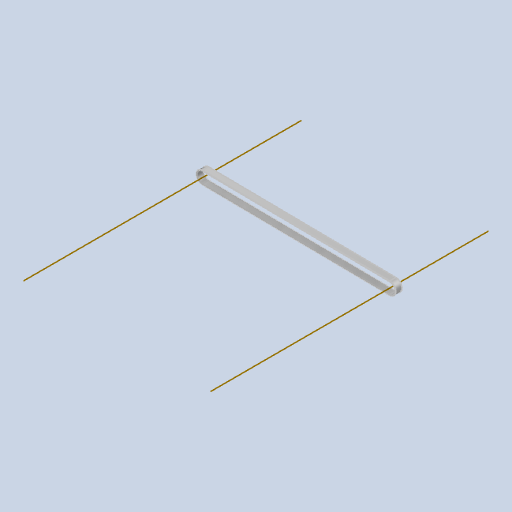
# Autodesk Inventor part: Synchronous Belt
Saved by Autodesk Inventor 2023 (Build 270158000, 158)
## iProperties
Created: 2022-10-18
Part Number: Synchronous Belt
Material: Rubber
Document SubType Name: Modeling
Designer: klebe
Density: 1 g/cm^3
Appearance: Rubber - Black - Version 1.1
CustomPartVersion: 1
Author: klebe
Autodesk Inventor part; units mm, degrees
sketch "Sketch Path" plane through (0, 0, 0) normal (0, 0, 1) x (1, 0, 0)
  arc A0 (0.0703, 6.0634) -> (-0.0703, -6.0634) centre (0, 0) ccw
  arc A1 (196.5726, -8.3439) -> (196.7132, 3.7829) centre (196.6429, -2.2805) ccw
  line L0 (196.5726, -8.3439) -> (-0.0703, -6.0634)
  line L1 (0.0703, 6.0634) -> (196.7132, 3.7829)
  constraints: 4 end point, 2 point on circle, 1 centre point, 3 other
ref_plane "Cross Section Plane" through (-0.0703, -6.0634, 0) normal (0.9999, -0.0116, 0) x (0, 0, 1)
ref_plane "Work Plane2" through (0, 0, 0) normal (-1, 0, 0) x (0, 0, 1)
ref_plane "Work Plane3" through (196.6429, -2.2805, 0) normal (-0.9995, 0.032, 0) x (0, 0, 1)
sketch "Cross Section" plane through (-0.0703, -6.0634, 0) normal (0.9999, -0.0116, 0) x (0, 0, 1)
  line L0 (-3.175, 0.508) -> (3.175, 0.508)
  line L1 (3.175, 0.508) -> (3.175, -0.254)
  line L2 (3.175, -0.254) -> (-3.175, -0.254)
  line L3 (-3.175, -0.254) -> (-3.175, 0.508)
  line L4 (-3.175, 0) -> (3.175, 0) construction
  point P0 (0, 0)
  point P1 (0, 0)
  dimension "d0" = 6.35
  dimension "d4" = 0.254
  dimension "d5" = 0.508
  constraints: 10 end point, 2 parallel, 2 point on line, 1 coincident, 1 horizontal, 1 midpoint, 1 perpendicular, 1 other
  measures "d0" distance between parallel lines of L1 L3
  measures "d4" distance between parallel lines of L2 L4
  measures "d5" distance between parallel lines of L4 L0
sweep "Belt" add profiles "Cross Section" path "Sketch Path"
equation "\"d0\" = da_B"
equation "\"d4\" = da_a"
equation "\"d5\" = da_a2"
equation "\"da_B\" = 6.35"
equation "\"da_pb\" = 3.175"
equation "\"da_L\" = 431.41219"
equation "\"da_a\" = 0.254"
equation "\"da_S\" = 1.7272"
equation "\"da_Beta\" = 25deg"
equation "\"da_Ht\" = 0.762"
equation "\"da_H\" = 1.524"
equation "\"da_a2\" = 0.508"
body "Solid1"
